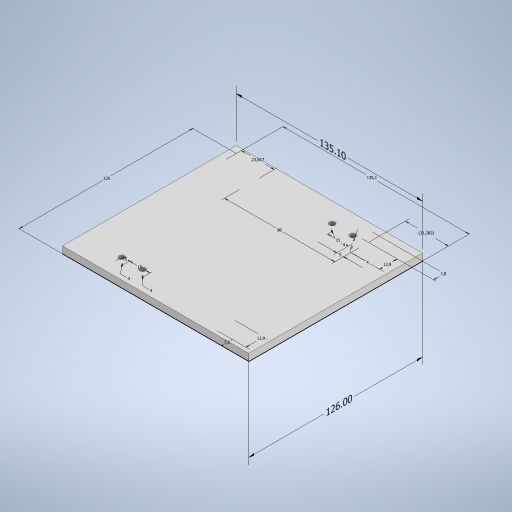
# Autodesk Inventor part: PiattoBilancia
Saved by Autodesk Inventor 2024.2 (Build 282272000, 272)
## iProperties
Created: 2025-05-27
Part Number: PiattoBilancia
Material: Generico
Document SubType Name: Modeling
Designer: zagom
Density: 1 g/cm^3
Appearance: Default
Author: zagom
Autodesk Inventor part; units mm, degrees
ref_plane "YZ Plane" through (0, 0, 0) normal (1, 0, 0) x (0, 1, 0)
ref_plane "XZ Plane" through (0, 0, 0) normal (0, 1, 0) x (-1, 0, 0)
ref_plane "XY Plane" through (0, 0, 0) normal (0, 0, 1) x (1, 0, 0)
sketch "Schizzo1" plane through (0, 0, 0) normal (0, 1, 0) x (-1, 0, 0)
  line L0 (-67.55, 63) -> (67.55, 63)
  line L1 (67.55, 63) -> (67.55, -63)
  line L2 (67.55, -63) -> (-67.55, -63)
  line L3 (-67.55, -63) -> (-67.55, 63)
  line L4 (-67.55, 63) -> (67.55, -63) construction
  line L5 (67.55, 63) -> (-67.55, -63) construction
  line L6 (67.55, -55.2) -> (43.733, -55.2) construction
  line L7 (43.733, -55.2) -> (-36.267, -55.2) construction
  line L8 (-36.267, -55.2) -> (-36.267, -42.3) construction
  line L9 (-36.267, -42.3) -> (43.733, -42.3) construction
  line L10 (43.733, -42.3) -> (43.733, -55.2) construction
  line L11 (-36.267, 63) -> (-36.267, 55.2) construction
  line L12 (-36.267, 55.2) -> (43.733, 55.2) construction
  line L13 (43.733, 55.2) -> (43.733, 42.3) construction
  line L14 (43.733, 42.3) -> (-36.267, 42.3) construction
  line L15 (-36.267, 42.3) -> (-36.267, 55.2) construction
  line L16 (-36.267, -48.75) -> (-31.267, -48.75) construction
  circle A0 centre (-31.267, -48.75) radius 2
  line L17 (-31.267, -48.75) -> (-16.267, -48.75) construction
  circle A1 centre (-16.267, -48.75) radius 2
  line L18 (43.733, 48.75) -> (38.733, 48.75) construction
  circle A2 centre (38.733, 48.75) radius 2
  line L19 (38.733, 48.75) -> (23.733, 48.75) construction
  circle A3 centre (23.733, 48.75) radius 2
  line L20 (-31.267, -63) -> (-31.267, -55.2) construction
  point P0 (0, 0)
  dimension "d0" = 135.1
  dimension "d1" = 126
  dimension "d18" = 23.817
  dimension "d19" = 80
  dimension "d20" = 12.9
  dimension "d21" = 7.8
  dimension "d22" = 12.9
  dimension "d23" = 5
  dimension "d24" = 31.283
  dimension "d26" = 4
  dimension "d27" = 15
  dimension "d28" = 4
  dimension "d37" = 5
  dimension "d38" = 4
  dimension "d39" = 15
  dimension "d40" = 4
  dimension "d55" = 7.8
  constraints: 42 end point, 8 coincident, 8 horizontal, 6 parallel, 4 centre point, 4 midpoint, 4 point on line, 3 perpendicular, 2 vertical
  measures "d0" distance of L1.end L2.end
  measures "d1" distance of L0.end L1.end
  measures "d18" distance of L6.start L6.end
  measures "d19" distance of L8.end L9.end
  measures "d20" distance of L7.end L8.end
  measures "d21" distance of L11.start L11.end
  measures "d22" distance of L14.end L11.end
  measures "d23" distance of L16.start L16.end
  measures "d24" distance between parallel lines of L3 L8
  measures "d26" diameter of A0
  measures "d27" distance of L17.start L17.end
  measures "d28" diameter of A1
  measures "d37" distance of L18.start L18.end
  measures "d38" diameter of A2
  measures "d39" distance of L19.start L19.end
  measures "d40" diameter of A3
  measures "d55" distance of L20.start L20.end
extrude "Estrusione1" add sketch "Schizzo1" along normal blind 5 contours L0 L1 L2 L3 | A0 | A1 | A2 | A3
hole "Foro3" at (16.267, 0, -48.75) at (31.267, 0, -48.75) at (-23.733, 0, 48.75) at (-38.733, 0, 48.75) direction (0, 1, 0) diameter 4 depth 10 countersink diameter 6 countersink angle 90
